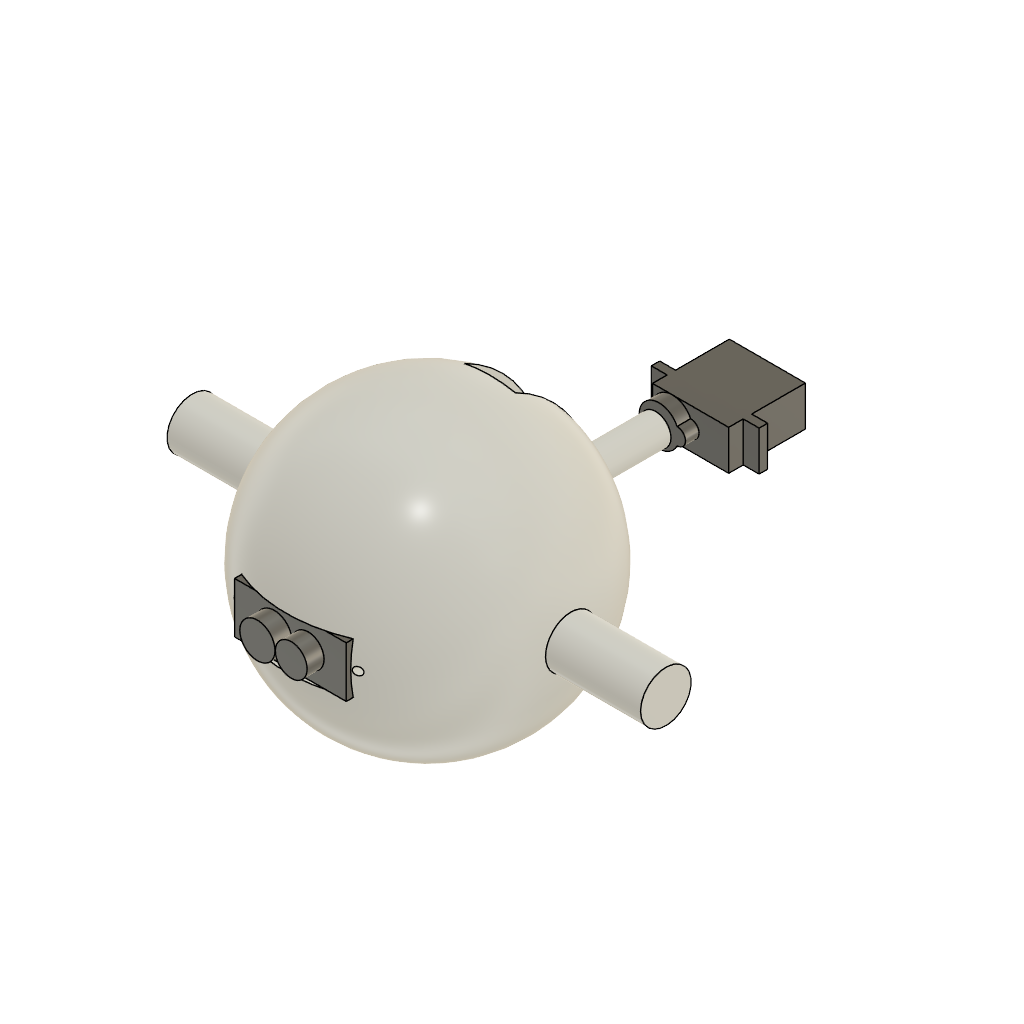
Eye Casing (Autodesk Fusion 360 design; units mm, degrees)
part number: 2026-09-18-12-27-33-073
Autodesk Fusion 360 part; units mm, degrees
note: some values were not read from the file. Chosen so that the rebuilt part matches the saved one: which pieces of a blend or face edit are solid. Set by a fixed rule: which sketch regions a step uses.
sketch "Sketch5" plane through (0, 0, 0) normal (0, 0, 1) x (1, 0, 0)
  line L0 (16.5, 7.5) -> (-16.5, 7.5)
  line L1 (-16.5, 7.5) -> (-16.5, -7.5)
  line L2 (-16.5, -7.5) -> (16.5, -7.5)
  line L3 (16.5, -7.5) -> (16.5, 7.5)
  line L4 (16.5, 7.5) -> (-16.5, -7.5) construction
  line L5 (-16.5, 7.5) -> (16.5, -7.5) construction
  line L6 (21, 7.5) -> (-21, 7.5) construction
  line L7 (-21, 7.5) -> (-21, -7.5) construction
  line L8 (-21, -7.5) -> (21, -7.5) construction
  line L9 (21, -7.5) -> (21, 7.5) construction
  line L10 (21, 7.5) -> (-21, -7.5) construction
  line L11 (-21, 7.5) -> (21, -7.5) construction
  line L12 (18, -7.5) -> (-18, -7.5) construction
  line L13 (-18, -7.5) -> (-18, 7.5) construction
  line L14 (-18, 7.5) -> (18, 7.5) construction
  line L15 (18, 7.5) -> (18, -7.5) construction
  line L16 (18, -7.5) -> (-18, 7.5) construction
  line L17 (-18, -7.5) -> (18, 7.5) construction
  circle A0 centre (-18, 0) radius 1.175
  circle A1 centre (18, 0) radius 1.175
  line L18 (-16.5, 7.5) -> (-21, 0)
  line L19 (-16.5, -7.5) -> (-21, 0)
  line L20 (16.5, 7.5) -> (21, 0)
  line L21 (21, 0) -> (16.5, -7.5)
  dimension "d6" = 33
  dimension "d7" = 15
  dimension "d8" = 42
  dimension "d9" = 15
  dimension "d12" = 36
  dimension "d13" = 15
  dimension "d14" = 2.35
  dimension "d15" = 2.35
  constraint horizontal L0
  constraint perpendicular L0 L1
  constraint parallel L0 L2
  constraint parallel L1 L3
  constraint coincident L4 origin
  constraint coincident L5 origin
  constraint horizontal L6
  constraint perpendicular L6 L7
  constraint parallel L6 L8
  constraint parallel L7 L9
  constraint coincident L10 origin
  constraint coincident L11 origin
  constraint horizontal L12
  constraint perpendicular L12 L13
  constraint parallel L12 L14
  constraint parallel L13 L15
  constraint coincident L16 origin
  constraint coincident L17 origin
  constraint midpoint L13 A0.centre
  constraint midpoint L7 L18.end
  constraint midpoint L9 L20.end
  measures "d6" distance of L1.end L2.end
  measures "d7" distance of L0.end L1.end
  measures "d8" distance of L7.end L8.end
  measures "d9" distance of L6.end L7.end
  measures "d12" distance of L13.end L14.end
  measures "d13" distance of L12.end L13.end
  measures "d14" diameter of A0
  measures "d15" diameter of A1
extrude "Extrude2" add sketch "Sketch5" along normal blind 5 contours L3 L20 L21 | L1 L18 L19 makes body 1 at (-16.5, 2.5, 1.6667) makes body 2 at (16.5, -2.5, 1.6667)
extrude "Extrude3" add sketch "Sketch5" along normal blind 11 separate body contours L0 L1 L2 L3 makes body 3
sketch "Sketch7" plane through (0, 0, 11) normal (0, 0, 1) x (-1, 0, 0)
  line L0 (-16.5, 7.5) -> (-16.5, -7.5)
  line L1 (-16.5, -7.5) -> (16.5, -7.5)
  line L2 (16.5, -7.5) -> (16.5, 7.5)
  line L3 (16.5, 7.5) -> (-16.5, 7.5)
  line L4 (-9.95, 2.5) -> (9.95, 2.5)
  line L5 (9.95, 2.5) -> (9.95, -2.5)
  line L6 (9.95, -2.5) -> (-9.95, -2.5)
  line L7 (-9.95, -2.5) -> (-9.95, 2.5)
  line L8 (-9.95, 2.5) -> (9.95, -2.5) construction
  line L9 (9.95, 2.5) -> (-9.95, -2.5) construction
  circle A0 centre (-4.75, 0) radius 5.2
  line L10 (9.95, 0) -> (-9.95, 0) construction
  circle A1 centre (5.25, 0) radius 4.7
  dimension "d20" = 19.9
  dimension "d21" = 5
  dimension "d22" = 10.4
  dimension "d23" = 9.4
  constraint horizontal L4
  constraint perpendicular L4 L5
  constraint parallel L4 L6
  constraint parallel L5 L7
  constraint coincident L8 origin
  constraint coincident L9 origin
  constraint tangent L7 A0
  constraint midpoint L5 L10.start
  constraint midpoint L7 L10.end
  constraint coincident A0.centre L10
  constraint coincident L10 A1.centre
  constraint tangent L5 A1
  measures "d20" distance of L5.end L6.end
  measures "d21" distance of L4.end L5.end
  measures "d22" diameter of A0
  measures "d23" diameter of A1
extrude "Extrude4" add sketch "Sketch7" along normal blind 5 contours L4 A0 | L4 L6 A0 | L6 A0 | L4 A1 | L4 L6 A1 | L6 A1 bodies 3
move_body "Move3" bodies 1 2 3 to x (-1, 0, 0) y (0, 1, 0) z (0, 0, -1) at (0, 0, 0)
sketch "Sketch11" plane through (0, 0, 0) normal (0, 0, 1) x (1, 0, 0)
  line L0 (0, 17.5) -> (0, 102.5)
  arc A0 (0, 20) -> (0, 100) centre (0, 60) ccw
  arc A1 (0, 17.5) -> (0, 102.5) centre (0, 60) ccw
  dimension "d28" = 80
  dimension "d29" = 85
  constraint concentric A0 A1
  constraint perpendicular L0 A1
  constraint coincident L0 A0.end
  constraint coincident L0 A0.start
  measures "d28" diameter of A0
  measures "d29" diameter of A1
revolve "Revolve1" add sketch "Sketch11" angle 360 about axis through (0, 1.75, 0) along (0, 1, 0) separate body contours L0 A0 A1 makes body 4
move_body "Move5" bodies 4 to x (1, 0, 0) y (0, 1, 0) z (0, 0, 1) at (0, -60, 32)
ref_plane "WorkPlane1" through (0, 0, 75) normal (0, 0, 1) x (1, 0, 0)
sketch "Sketch12" plane through (0, 0, 75) normal (0, 0, 1) x (1, 0, 0)
  line L0 (7.5, 42.5) -> (-7.5, 42.5)
  line L1 (-7.5, 42.5) -> (-7.5, -42.5)
  line L2 (-7.5, -42.5) -> (7.5, -42.5)
  line L3 (7.5, -42.5) -> (7.5, 42.5)
  line L4 (7.5, 42.5) -> (-7.5, -42.5) construction
  line L5 (-7.5, 42.5) -> (7.5, -42.5) construction
  dimension "d33" = 15
  dimension "d34" = 85
  constraint horizontal L0
  constraint perpendicular L0 L1
  constraint parallel L0 L2
  constraint parallel L1 L3
  constraint coincident L4 origin
  constraint coincident L5 origin
  measures "d33" distance of L1.end L2.end
  measures "d34" distance of L0.end L1.end
extrude "Extrude5" cut sketch "Sketch12" against normal blind 25 bodies 4
move_body "Move6" bodies 3 1 4 2 to x (1, 0, 0) y (0, 0, -1) z (0, 1, 0) at (0, -20, 0)
move_face "MoveFace2" to x (1, 0, 0) y (0, 1, 0) z (0, 0, 1) at (0, -0.5, 0) 1 faces at (40.2932, 1.9538, 9.0434) on bodies 4
sketch "Sketch13" plane through (0, -31, 0) normal (0, -1, 0) x (1, 0, 0)
  circle A0 centre (-4.75, 0) radius 5.2
  circle A1 centre (5.25, 0) radius 4.7
  line L0 (-16.5, 7.5) -> (-16.5, -7.5)
  line L1 (-16.5, -7.5) -> (16.5, -7.5)
  line L2 (16.5, -7.5) -> (16.5, 7.5)
  line L3 (16.5, 7.5) -> (-16.5, 7.5)
  circle A2 centre (-18, 0) radius 1.175
  circle A3 centre (18, 0) radius 1.175
  dimension "d38" = 2.35
  dimension "d39" = 2.35
  measures "d38" diameter of A2
  measures "d39" diameter of A3
extrude "Extrude6" cut sketch "Sketch13" against normal blind 10 contours A2 | A3 bodies 4
ref_plane "WorkPlane2" through (0, -31, 0) normal (0, 1, 0) x (0, 0, 1)
sketch "Sketch14" plane through (0, -31, 0) normal (0, 1, 0) x (1, 0, 0)
  line L0 (16.5, 7.5) -> (-16.5, 7.5)
  line L1 (-16.5, 7.5) -> (-16.5, -7.5)
  line L2 (-16.5, -7.5) -> (16.5, -7.5)
  line L3 (16.5, -7.5) -> (16.5, 7.5)
  line L4 (16.5, 7.5) -> (-16.5, -7.5) construction
  line L5 (-16.5, 7.5) -> (16.5, -7.5) construction
  dimension "d44" = 33
  dimension "d45" = 15
  constraint horizontal L0
  constraint perpendicular L0 L1
  constraint parallel L0 L2
  constraint parallel L1 L3
  constraint coincident L4 origin
  constraint coincident L5 origin
  measures "d44" distance of L1.end L2.end
  measures "d45" distance of L0.end L1.end
extrude "Extrude7" cut sketch "Sketch14" along normal blind 17 bodies 4
combine "Combine1" operation add target body 1 tool bodies 2 3
move_body "Move8" bodies 4 to x (1, 0, 0) y (0, 1, 0) z (0, 0, 1) at (0, -12, 0)
sketch "Sketch15" plane through (0, 0, 0) normal (1, 0, 0) x (0, 1, 0)
  circle A0 centre (0, 0) radius 7.5
  dimension "d48" = 15
  constraint coincident A0.centre origin
  measures "d48" diameter of A0
extrude "Extrude8" cut sketch "Sketch15" along normal mid plane 200 bodies 4
sketch "Sketch16" plane through (0, 0, 0) normal (0, 0, 1) x (1, 0, 0)
  line L0 (-15, 15) -> (15, 15)
  line L1 (15, 15) -> (15, -15)
  line L2 (15, -15) -> (-15, -15)
  line L3 (-15, -15) -> (-15, 15)
  line L4 (-15, 15) -> (15, -15) construction
  line L5 (15, 15) -> (-15, -15) construction
  dimension "d51" = 30
  dimension "d52" = 30
  constraint horizontal L0
  constraint perpendicular L0 L1
  constraint parallel L0 L2
  constraint parallel L1 L3
  constraint coincident L4 origin
  constraint coincident L5 origin
  measures "d51" distance of L1.end L2.end
  measures "d52" distance of L0.end L1.end
extrude "Extrude9" add sketch "Sketch16" along normal mid plane 30 separate body makes body 5
shell "Shell1" thickness 3 removed faces 0 bodies 5
extrude "Extrude10" cut 1 faces at (5, 15, 5) along direction (0, -1, 0) blind 2 on bodies 5 bodies 5
extrude "Extrude11" add 1 faces at (5, 13, 5) along direction (0, 1, 0) blind 2 on bodies 5 bodies 5
sketch "Sketch17" plane through (15, 0, 0) normal (1, 0, 0) x (0, 1, 0)
  line L0 (15, 15) -> (-15, 15)
  line L1 (-15, 15) -> (-15, -15)
  line L2 (-15, -15) -> (15, -15)
  line L3 (15, -15) -> (15, 15)
  circle A0 centre (0, 0) radius 7.5
  dimension "d60" = 15
  constraint coincident A0.centre origin
  measures "d60" diameter of A0
extrude "Extrude12" add sketch "Sketch17" along normal blind 100 contours A0 bodies 5
sketch "Sketch19" plane through (-15, 0, 0) normal (-1, 0, 0) x (0, -1, 0)
  line L0 (-15, -15) -> (15, -15)
  line L1 (15, -15) -> (15, 15)
  line L2 (15, 15) -> (-15, 15)
  line L3 (-15, 15) -> (-15, -15)
  circle A0 centre (0, 0) radius 7.5
  dimension "d63" = 15
  constraint coincident A0.centre origin
  measures "d63" diameter of A0
extrude "Extrude13" add sketch "Sketch19" along normal blind 100 contours A0 bodies 5
extrude "Extrude14" cut 1 faces at (-115, -1.9158, 2.8099) along direction (1, 0, 0) blind 45 on bodies 5 bodies 5
extrude "Extrude15" cut 1 faces at (115, 0.4732, -2.8016) along direction (-1, 0, 0) blind 45 on bodies 5 bodies 5
ref_plane "WorkPlane3" through (0, -35, 0) normal (0, 1, 0) x (0, 0, 1)
sketch "Sketch20" plane through (0, -35, 0) normal (0, 1, 0) x (1, 0, 0)
  line L0 (16.5, 7.5) -> (-16.5, 7.5) construction
  line L1 (-16.5, 7.5) -> (-16.5, -7.5) construction
  line L2 (-16.5, -7.5) -> (16.5, -7.5) construction
  line L3 (16.5, -7.5) -> (16.5, 7.5) construction
  line L4 (16.5, 7.5) -> (-16.5, -7.5) construction
  line L5 (-16.5, 7.5) -> (16.5, -7.5) construction
  line L6 (-16.5, 7.5) -> (16.5, 7.5)
  line L7 (16.5, 7.5) -> (16.5, 11.5)
  line L8 (16.5, 11.5) -> (-16.5, 11.5)
  line L9 (-16.5, 11.5) -> (-16.5, 7.5)
  dimension "d72" = 33
  dimension "d73" = 15
  dimension "d74" = 33
  dimension "d75" = 4
  constraint horizontal L0
  constraint perpendicular L0 L1
  constraint parallel L0 L2
  constraint parallel L1 L3
  constraint coincident L4 origin
  constraint coincident L5 origin
  constraint horizontal L6
  constraint vertical L7
  constraint horizontal L8
  constraint vertical L9
  measures "d72" distance of L1.end L2.end
  measures "d73" distance of L0.end L1.end
  measures "d74" distance of L0.end L0.start
  measures "d75" distance of L0.end L8.end
extrude "Extrude16" add sketch "Sketch20" against normal blind 2 bodies 4
extrude "Extrude17" add 1 faces at (4.4064, -37, -9.3631) along direction (0, -1, 0) blind 2 on bodies 4 bodies 4
extrude "Extrude18" add 1 faces at (-0.4182, -39, -8.3318) along direction (0, -1, 0) blind 1 on bodies 4 bodies 4
extrude "Extrude19" add 1 faces at (5.1935, -35, -8.8333) along direction (0, 1, 0) blind 10 on bodies 4 bodies 4
extrude "Extrude20" cut 1 faces at (5.1935, -25, -8.8333) along direction (0, -1, 0) blind 0.658 on bodies 4 bodies 4
move_body "Move9" bodies 1 to x (1, 0, 0) y (0, 1, 0) z (0, 0, 1) at (0, -10, 0)
sketch "Sketch21" plane through (0, 0, 0) normal (0, 0, 1) x (1, 0, 0)
  line L0 (-11.25, 5.9) -> (11.25, 5.9)
  line L1 (11.25, 5.9) -> (11.25, -5.9)
  line L2 (11.25, -5.9) -> (-11.25, -5.9)
  line L3 (-11.25, -5.9) -> (-11.25, 5.9)
  line L4 (-11.25, 5.9) -> (11.25, -5.9) construction
  line L5 (11.25, 5.9) -> (-11.25, -5.9) construction
  dimension "d86" = 22.5
  dimension "d87" = 11.8
  constraint horizontal L0
  constraint perpendicular L0 L1
  constraint parallel L0 L2
  constraint parallel L1 L3
  constraint coincident L4 origin
  constraint coincident L5 origin
  measures "d86" distance of L1.end L2.end
  measures "d87" distance of L0.end L1.end
extrude "Extrude21" add sketch "Sketch21" along normal blind 22.7 separate body makes body 6
ref_plane "WorkPlane4" through (0, 0, 15.9) normal (0, 0, 1) x (1, 0, 0)
sketch "Sketch23" plane through (0, 0, 15.9) normal (0, 0, 1) x (1, 0, 0)
  line L0 (-15.95, 5.9) -> (15.95, 5.9)
  line L1 (15.95, 5.9) -> (15.95, -5.9)
  line L2 (15.95, -5.9) -> (-15.95, -5.9)
  line L3 (-15.95, -5.9) -> (-15.95, 5.9)
  line L4 (-15.95, 5.9) -> (15.95, -5.9) construction
  line L5 (15.95, 5.9) -> (-15.95, -5.9) construction
  dimension "d92" = 31.9
  dimension "d93" = 11.8
  constraint horizontal L0
  constraint perpendicular L0 L1
  constraint parallel L0 L2
  constraint parallel L1 L3
  constraint coincident L4 origin
  constraint coincident L5 origin
  measures "d92" distance of L1.end L2.end
  measures "d93" distance of L0.end L1.end
extrude "Extrude22" add sketch "Sketch23" along normal blind 2.5 bodies 6
sketch "Sketch24" plane through (0, 0, 22.7) normal (0, 0, 1) x (-1, 0, 0)
  line L0 (11.25, 5.9) -> (-11.25, 5.9)
  line L1 (-11.25, 5.9) -> (-11.25, -5.9)
  line L2 (-11.25, -5.9) -> (11.25, -5.9)
  line L3 (11.25, -5.9) -> (11.25, 5.9)
  circle A0 centre (5.35, 0) radius 5.9
  line L4 (11.25, -5.9) -> (11.25, 5.9) construction
  circle A1 centre (0, 0) radius 2.5
  dimension "d96" = 11.8
  dimension "d97" = 5
  constraint coincident L2.end L3.start
  constraint coincident L0.start L3.end
  constraint tangent A0 L4
  constraint coincident A1.centre origin
  measures "d96" diameter of A0
  measures "d97" diameter of A1
extrude "Extrude23" add sketch "Sketch24" along normal blind 4 contours A0 A1 | A0 A1 | A0 A1 bodies 6
sketch "Sketch25" plane through (0, 0, 26.7) normal (0, 0, 1) x (-1, 0, 0)
  arc A0 (0.0058, -2.5) -> (0.0058, 2.5) centre (5.35, 0) ccw
  arc A1 (0.0058, 2.5) -> (0.0058, -2.5) centre (0, 0) ccw
  circle A2 centre (5.35, 0) radius 2.3
  dimension "d100" = 4.6
  constraint concentric A0 A2
  measures "d100" diameter of A2
extrude "Extrude24" add sketch "Sketch25" along normal blind 3.2 contours A2 bodies 6
move_body "Move10" bodies 6 to x (1, 0, 0) y (0, 0, 1) z (0, -1, 0) at (5, 125, 0)
move_body "Move11" bodies 6 to x (1, 0, 0) y (0, 1, 0) z (0, 0, 1) at (0, -30, 0)
extrude "Extrude25" cut 1 faces at (5, 15, 5) along direction (0, -1, 0) blind 3 on bodies 5 bodies 5
extrude "Extrude26" add 1 faces at (-14, 12, -4) along direction (0, 1, 0) blind 3 on bodies 5 bodies 5
sketch "Sketch27" plane through (0, 0, 0) normal (0, 0, 1) x (1, 0, 0)
  circle A0 centre (0, 0) radius 4.5
  dimension "d108" = 9
  constraint coincident A0.centre origin
  measures "d108" diameter of A0
extrude "Extrude27" add sketch "Sketch27" along normal blind 50 separate body makes body 7
sketch "Sketch28" plane through (0, 0, 50) normal (0, 0, 1) x (-1, 0, 0)
  circle A0 centre (0, 0) radius 4.5
  circle A1 centre (0, 0) radius 2.35
  dimension "d111" = 4.7
  constraint coincident A0.centre A1.centre
  measures "d111" diameter of A1
extrude "Extrude28" cut sketch "Sketch28" against normal blind 3.2 contours A1 bodies 7
move_body "Move12" bodies 7 to x (1, 0, 0) y (0, 0, -1) z (0, 1, 0) at (0, 0, 0)
move_body "Move13" bodies 7 to x (1, 0, 0) y (0, 1, 0) z (0, 0, 1) at (0, 17, 0)
equation "d92 = 22.5 mm + ( 2 * 4.7 ) * 1 mm"
named bodies: "Sonar", "Eye casing", "Internal Axis/Gear chamber", "Servo", "Shaft"
